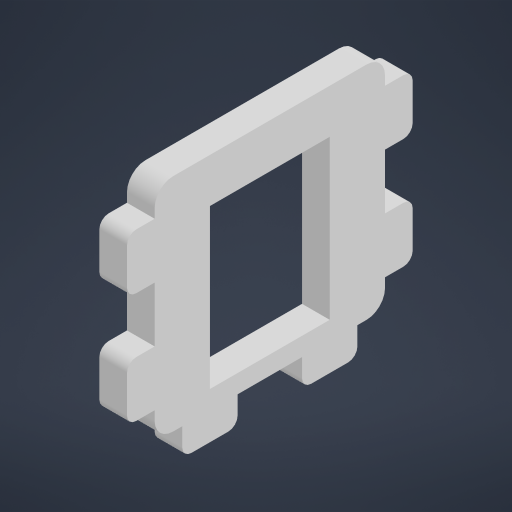
# Autodesk Inventor part: FacePlate
Saved by Autodesk Inventor 2023 (Build 270158000, 158)
## iProperties
Created: 2023-03-14
Part Number: FacePlate
Material: Generic
Document SubType Name: Modeling
Designer: Matt
Density: 1 g/cm^3
Appearance: Default
Author: Matt
Autodesk Inventor part; units mm, degrees
ref_plane "YZ Plane" through (0, 0, 0) normal (1, 0, 0) x (0, 1, 0)
ref_plane "XZ Plane" through (0, 0, 0) normal (0, 1, 0) x (-1, 0, 0)
ref_plane "XY Plane" through (0, 0, 0) normal (0, 0, 1) x (1, 0, 0)
sketch "Sketch1" plane through (0, 0, 0) normal (1, 0, 0) x (0, 1, 0)
  line L0 (0, 0) -> (24, 0)
  line L1 (24, 0) -> (24, -25)
  line L2 (24, -25) -> (0, -25)
  line L3 (0, -25) -> (0, 0)
  dimension "d0" = 24
  dimension "d1" = 25
  constraints: 8 end point, 2 parallel, 1 horizontal, 1 perpendicular
  measures "d0" distance of L1.end L2.end
  measures "d1" distance of L0.end L1.end
extrude "Front Plate" add sketch "Sketch1" along normal blind 3
sketch "Sketch2" plane through (3, 0, 0) normal (1, 0, 0) x (0, 0, -1)
  line L0 (0, 24) -> (0, 0) projected
  line L1 (0, 21) -> (-3, 21)
  line L2 (-3, 21) -> (-3, 15)
  line L3 (-3, 15) -> (0, 15)
  line L4 (0, 15) -> (0, 21)
  line L5 (25, 24) -> (0, 24) projected
  line L6 (12.5, -1.4018) -> (12.5, 28.9484)
  line L7 (29.0475, 12) -> (-9.9529, 12)
  line L8 (0, 3) -> (-3, 3)
  line L9 (-3, 3) -> (-3, 9)
  line L10 (-3, 9) -> (0, 9)
  line L11 (0, 9) -> (0, 3)
  line L12 (0, 0) -> (25, 0) projected
  line L13 (3, 0) -> (9, 0)
  line L14 (9, 0) -> (9, -3)
  line L15 (9, -3) -> (3, -3)
  line L16 (3, -3) -> (3, 0)
  line L17 (25, 21) -> (28, 21)
  line L18 (28, 21) -> (28, 15)
  line L19 (28, 15) -> (25, 15)
  line L20 (25, 15) -> (25, 21)
  line L21 (25, 3) -> (28, 3)
  line L22 (28, 3) -> (28, 9)
  line L23 (28, 9) -> (25, 9)
  line L24 (25, 9) -> (25, 3)
  line L25 (22, 0) -> (16, 0)
  line L26 (16, 0) -> (16, -3)
  line L27 (16, -3) -> (22, -3)
  line L28 (22, -3) -> (22, 0)
  point P0 (0, 9)
  point P1 (9, 0)
  point P2 (0, 15)
  dimension "d4" = 3
  dimension "d5" = 6
  dimension "d6" = 3
  dimension "d7" = 3
  dimension "d8" = 6
  dimension "d9" = 3
  constraints: 52 end point, 16 symmetric about line, 4 parallel, 3 horizontal, 2 perpendicular, 2 point on line, 1 vertical
  measures "d4" distance of L3.end L2.end
  measures "d5" distance of L1.end L2.end
  measures "d6" distance between parallel lines of L5 L1
  measures "d7" distance of L13.end L14.end
  measures "d8" distance of L14.end L15.end
  measures "d9" distance between parallel lines of L0 L16
extrude "Pegs" add sketch "Sketch2" against normal blind 3 contours L12 L28 L27 L26 | L0 L3 L2 L1 | L0 L8 L9 L10 | L14 L15 L16 L12 | L17 L18 L19 L20 | L24 L23 L22 L21
sketch "Sketch3" plane through (3, 0, 0) normal (1, 0, 0) x (0, 0, -1)
  line L0 (6, 19.2) -> (19, 19.2)
  line L1 (19, 19.2) -> (19, 2)
  line L2 (19, 2) -> (6, 2)
  line L3 (6, 2) -> (6, 19.2)
  line L4 (25, 9) -> (25, 15) projected
  line L5 (0, 15) -> (0, 9) projected
  line L6 (25, 24) -> (0, 24) projected
  line L7 (9, 0) -> (16, 0) projected
  point P0 (0, 0)
  dimension "d12" = 6
  dimension "d13" = 6
  dimension "d14" = 4.8
  dimension "d15" = 2
  constraints: 8 end point, 2 parallel, 1 horizontal, 1 perpendicular
  measures "d12" distance between parallel lines of L4 L1
  measures "d13" distance between parallel lines of L5 L3
  measures "d14" distance between parallel lines of L6 L0
  measures "d15" distance between parallel lines of L7 L2
extrude "Camera CutOut" cut sketch "Sketch3" against normal blind 3
fillet "PiCam Corner Radius" radius 2 4 edges at (1.5, 24, 0) (1.5, 24, -25) (1.5, 0, -25) (1.5, 0, 0)
fillet "Peg Fillet" radius 1 12 edges at (1.5, 21, 3) (1.5, 15, 3) (1.5, 9, 3) (1.5, 3, 3) (1.5, -3, -3) (1.5, -3, -9) (1.5, -3, -16) (1.5, -3, -22) (1.5, 3, -28) (1.5, 9, -28) (1.5, 15, -28) (1.5, 21, -28)
equation "\"d0\" = CameraHeight"
equation "\"d1\" = CameraWidth"
equation "\"d2\" = Acrylic"
equation "\"d4\" = Acrylic"
equation "\"d5\" = 0.25 * CameraHeight"
equation "\"d7\" = Acrylic"
equation "\"d8\" = d5"
equation "\"d9\" = d6"
equation "\"d10\" = Acrylic"
equation "\"d13\" = d12"
equation "\"d16\" = Acrylic"
equation "\"CameraHeight\" = 24"
equation "\"CameraWidth\" = 25"
equation "\"Acrylic\" = 3"
body "Solid1"
